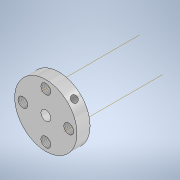
# Autodesk Inventor part: Планшайба D19
Saved by Autodesk Inventor 2020 (Build 240168000, 168)
## iProperties
Created: 2021-08-12
Part Number: Планшайба D19
Material: Типовые
Document SubType Name: Modeling
Designer: Антон
Density: 1 g/cm^3
Appearance: Алюминий — темный
Author: Антон
Autodesk Inventor part; units mm, degrees
ref_plane "YZ Plane" through (0, 0, 0) normal (1, 0, 0) x (0, 1, 0)
ref_plane "XZ Plane" through (0, 0, 0) normal (0, 1, 0) x (-1, 0, 0)
ref_plane "XY Plane" through (0, 0, 0) normal (0, 0, 1) x (1, 0, 0)
sketch "Эскиз1" plane through (0, 0, 0) normal (0, 0, 1) x (1, 0, 0)
  circle A0 centre (0, 0) radius 9.5
  dimension "d0" = 19
  constraints: 1 centre point, 1 coincident
  measures "d0" diameter of A0
extrude "Выдавливание1" add sketch "Эскиз1" along normal blind 4
sketch "Эскиз2" plane through (0, 0, 4) normal (0, 0, 1) x (1, 0, 0)
  circle A0 centre (0, 0) radius 7 construction
  line L0 (-7, 0) -> (7, 0) construction
  line L1 (0, 7) -> (0, -7) construction
  dimension "d3" = 14
  constraints: 4 end point, 2 coincident, 2 midpoint, 2 point on circle, 1 centre point, 1 perpendicular, 1 vertical
  measures "d3" diameter of A0
hole "Отверстие1" at (0, 7, 4) at (0, 0, 4) at (7, 0, 4) at (-7, 0, 4) at (0, -7, 4) direction (0, 0, -1) diameter 3 end through all
ref_plane "РабПлоскость1" through (7, 0, -23.1662) normal (-0.7071068, -0.7071068, 0) x (0, 0, 1)
sketch "Эскиз4" plane through (7, 0, -23.1662) normal (-0.7071068, -0.7071068, 0) x (0, 0, 1)
  line L0 (23.1662, 3.4497) -> (23.1662, 6.4497) projected
  line L1 (27.1662, 6.4497) -> (27.1662, 3.4497) projected
  line L2 (27.1662, -4.5503) -> (27.1662, 14.4497) projected
  line L3 (27.1662, 4.9497) -> (23.1662, 4.9497)
  point P0 (25.1662, 4.9497)
  constraints: 3 midpoint, 2 end point
hole "Отверстие2" at (3.5, 3.5, 2) direction (0.7071068, 0.7071068, 0) diameter 2 end through all
sketch "Эскиз5" plane through (3.5, 3.5, 2) normal (0.7071068, 0.7071068, 0) x (-0.7071068, 0.7071068, 0)
  circle A0 centre (0, 0) radius 1 projected
  point P0 (0, -2)
hole "Отверстие3" at (3.5, 3.5, 2) direction (-0.7071068, -0.7071068, 0) diameter 2 end up to face face through (0, 0, -23.1662) facing (0, 0, 1) round with radius 1.5 far side no
thread "Резьба1" size "M3x0.5" class "6H" standard "ANSI Metric M Profile" full length
thread "Резьба2" size "M3x0.5" class "6H" standard "ANSI Metric M Profile" full length
thread "Резьба3" size "M3x0.5" class "6H" standard "ANSI Metric M Profile" full length
thread "Резьба4" size "M3x0.5" class "6H" standard "ANSI Metric M Profile" full length
thread "Резьба5" size "M2x0.4" class "6H" standard "ANSI Metric M Profile" full length
